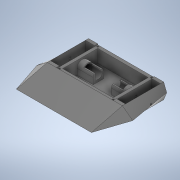
# Autodesk Inventor part: BodyWedgeV4
Saved by Autodesk Inventor 2020 (Build 240168000, 168)
## iProperties
Created: 2023-12-03
Part Number: BodyWedgeV4
Material: Thermoplastic Resin
Document SubType Name: Modeling
Designer: smz3rm
Density: 1.28 g/cm^3
Appearance: Smooth - Black
Mass: 334.957 g
Surface Area: 717.072 cm^2
Volume: 261.685 cm^3
Author: smz3rm
Autodesk Inventor part; units mm, degrees
ref_plane "YZ Plane" through (0, 0, 0) normal (1, 0, 0) x (0, 1, 0)
sketch "Sketch1" plane through (0, 0, 0) normal (0, 1, 0) x (-1, 0, 0)
  line L0 (55, 30) -> (-55, 30)
  line L1 (-55, 30) -> (-55, -30)
  line L2 (-55, -30) -> (55, -30)
  line L3 (55, -30) -> (55, 30)
  line L4 (55, 30) -> (-55, -30) construction
  line L5 (-55, 30) -> (55, -30) construction
  point P0 (0, 0)
  dimension "d0" = 110
  dimension "d1" = 60
  constraints: 12 end point, 2 midpoint, 2 parallel, 1 horizontal, 1 perpendicular
  measures "d0" distance of L2.end L1.end
  measures "d1" distance of L0.end L1.end
extrude "Extrusion1" add sketch "Sketch1" along normal blind 3
sketch "Sketch2" plane through (0, 3, 0) normal (0, 1, 0) x (1, 0, 0)
  line L0 (-55, 30) -> (-55, -30) projected
  line L1 (-55, -30) -> (55, -30) projected
  line L2 (55, -30) -> (55, 30) projected
  line L3 (55, 30) -> (-55, 30) projected
  line L4 (-49, 24) -> (-49, -24)
  line L5 (-49, -24) -> (49, -24)
  line L6 (49, -24) -> (49, 24)
  line L7 (49, 24) -> (-49, 24)
  point P0 (0, 0)
  dimension "d4" = 6
  constraints: 8 end point, 3 other
  measures "d4" distance between parallel lines of L3 L7
extrude "Extrusion2" add sketch "Sketch2" along normal blind 25.4125
sketch "Sketch3" plane through (-49, 3, 24) normal (1, 0, 0) x (0, 0, -1)
  line L0 (48, 0) -> (0, 0) projected
  line L1 (48, 0) -> (48, 25.4125) projected
  line L2 (0, 25.4125) -> (48, 25.4125) projected
  line L3 (0, 0) -> (0, 25.4125) projected
  circle A0 centre (38, 12) radius 8
  line L4 (54, -3) -> (-6, -3) projected
  circle A1 centre (38, 12) radius 10
  line L5 (48, 0) -> (48, 25.4125) projected
  line L6 (28, 12) -> (28, 0)
  point P0 (24, -3)
  point P1 (38, 22)
  point P2 (48, 12)
  dimension "d7" = 16
  dimension "d8" = 15
  dimension "d9" = 2
  constraints: 2 centre point, 2 end point, 2 point on circle, 2 tangent, 1 coincident, 1 point on line, 1 vertical
  measures "d7" diameter of A0
  measures "d8" distance from line of L4 A0.centre
  measures "d9" radial gap between concentric circles of A0 A1
extrude "Extrusion3" add sketch "Sketch3" along normal blind 11.25 contours L0 L6 A1 L1 | A1
sketch "Sketch4" plane through (-37.75, 3, 24) normal (1, 0, 0) x (0, 0, -1)
  line L0 (48, 12) -> (48, 0) projected
  arc A0 (48, 12) -> (28, 12) centre (38, 12) ccw projected
  line L1 (28, 12) -> (28, 0) projected
  line L2 (48, 0) -> (28, 0) projected
  circle A1 centre (38, 12) radius 8 projected
  circle A2 centre (38, 12) radius 7.75
  circle A3 centre (38, 12) radius 8 projected
  line L3 (48, 0) -> (28, 0) projected
  line L4 (32, 0) -> (32, 17.2915)
  line L5 (38, 19.75) -> (38, 4.25)
  line L6 (44, 0) -> (44, 17.2915)
  line L7 (32, 17.2915) -> (29.5147, 17.2915)
  arc A4 (48, 12) -> (28, 12) centre (38, 12) ccw projected
  line L8 (48, 12) -> (48, 0) projected
  line L9 (44, 17.2915) -> (46.4853, 17.2915)
  point P0 (24, -3)
  point P1 (48, 21)
  point P2 (39, 21)
  point P3 (44, 7.0946)
  point P4 (32, 7.0946)
  point P5 (44, 16.9054)
  point P6 (44, 0)
  point P7 (32, 16.9054)
  dimension "d13" = 15.5
  dimension "d14" = 15.5
  dimension "d15" = 12
  constraints: 10 end point, 4 point on circle, 2 horizontal, 2 symmetric about line, 1 centre point, 1 coincident, 1 perpendicular, 1 point on line, 1 vertical, 2 other
  measures "d13" diameter of A2
  measures "d14" distance of L5.start L5.end
  measures "d15" distance between parallel lines of L6 L4
extrude "Extrusion4" add sketch "Sketch4" along normal blind 20 contours L0 L2 L6 A1 L9 A0 | L2 L4 A1 L6 | L7 A1 L4 L2 L1 A0 | A1 L6 A2 | A1 L4 A2 L6 | L4 A2 A1 | L4 A2 picked at (37.1105, 4.2492)
sketch "Sketch13" plane through (-49, 15, -14) normal (1, 0, 0) x (0, 0, -1)
  circle A0 centre (0, 0) radius 2
  point P0 (-14, -15)
  dimension "d38" = 4
  constraints: 1 centre point
  measures "d38" diameter of A0
extrude "Extrusion13" cut sketch "Sketch13" against normal up to surface (6 mm away)
mirror "Mirror7" about plane through (0, 0, 0) normal (1, 0, 0) of "Extrusion3", "Extrusion4", "Extrusion13"
sketch "Sketch14" plane through (-55, 0, -30) normal (-1, 0, 0) x (0, 0, 1)
  circle A0 centre (16, 15) radius 2 projected
  line L0 (0, 0) -> (60, 0) projected
  line L1 (60, 0) -> (60, 28.4125) projected
  line L2 (0, 28.4125) -> (60, 28.4125) projected
  line L3 (0, 0) -> (0, 28.4125) projected
  line L4 (54, 28.4125) -> (54, 0)
  line L5 (0, 0) -> (60, 0) projected
  line L6 (54, 28.4125) -> (54, 30)
  line L7 (54, 30) -> (60, 30)
  line L8 (60, 30) -> (60, 28.4125)
  point P0 (30, 0)
  point P1 (54, 28.4125)
  point P2 (54, 28.4125)
  dimension "d74" = 1.5875
  constraints: 8 end point, 2 perpendicular, 2 vertical, 1 point on line
  measures "d74" distance of L4.start L6.end
extrude "Extrusion14" add sketch "Sketch14" along normal blind 17.78 contours L4 L2 L1 L0 | L6 L7 L8 L2
sketch "Sketch15" plane through (-55, 0, -30) normal (-1, 0, 0) x (0, 0, 1)
  line L0 (0, 28.4125) -> (54, 28.4125) projected
  line L1 (0, 0) -> (0, 28.4125) projected
  line L2 (0, 0) -> (54, 0) projected
  circle A0 centre (16, 15) radius 2 projected
  line L3 (0, 0) -> (0, 28.4125) projected
  line L4 (0, 28.4125) -> (-14, 28.4125)
  line L5 (-14, 28.4125) -> (-14, 0)
  line L6 (-14, 0) -> (0, 0)
  line L7 (54, 0) -> (54, 28.4125) projected
  point P0 (30, 0)
  dimension "d43" = 30
  constraints: 6 end point, 2 perpendicular, 1 horizontal
  measures "d43" distance from line of L5 A0.centre
extrude "Extrusion15" add sketch "Sketch15" against normal blind 6 contours L1 L6 L5 L4
sketch "Sketch16" plane through (0, 28.4125, 0) normal (0, 1, 0) x (1, 0, 0)
  line L0 (55, 30) -> (-49, 30) projected
  line L1 (-49, 44) -> (-49, 30) projected
  line L2 (-55, 44) -> (-49, 44) projected
  line L3 (-55, -24) -> (-55, 44) projected
  line L4 (-55, -30) -> (55, -30) projected
  line L5 (55, -30) -> (55, 30) projected
  line L6 (49, -24) -> (-49, -24) projected
  line L7 (-49, -24) -> (-49, 24) projected
  line L8 (-49, 24) -> (49, 24) projected
  line L9 (49, 24) -> (49, -24) projected
  line L10 (49, 24) -> (49, -24) projected
  line L11 (49, 24) -> (49, 30)
  line L12 (-49, 24) -> (49, 24) projected
  line L13 (55, 30) -> (-49, 30) projected
  line L14 (-49, 24) -> (-49, 30)
  line L15 (-55, -24) -> (-55, -30) projected
  point P0 (0, 0)
  constraints: 4 end point, 1 collinear, 1 point on line, 1 vertical
extrude "Extrusion16" cut sketch "Sketch16" against normal up to surface (25.4125 mm away) contours L11 L8 L14 L0
mirror "Mirror8" about plane through (0, 0, 0) normal (1, 0, 0) of "Extrusion15", "Extrusion14"
sketch "Sketch17" plane through (49, 0, -30) normal (0, 0, -1) x (-1, 0, 0)
  line L0 (0, 3) -> (0, 0) projected
  line L1 (0, 0) -> (98, 0) projected
  line L2 (98, 0) -> (98, 3) projected
  line L3 (98, 3) -> (0, 3) projected
  point P0 (49, 0)
extrude "Extrusion17" add sketch "Sketch17" along normal up to surface (14 mm away)
sketch "Sketch19" plane through (0, 0, 0) normal (0, -1, 0) x (1, 0, 0)
  line L0 (-55, -44) -> (-55, 24) projected
  line L1 (-55, -44) -> (55, -44) projected
  line L2 (55, 24) -> (55, -44) projected
  line L3 (72.78, 24) -> (72.78, 30) projected
  line L4 (72.78, 30) -> (-72.78, 30) projected
  line L5 (-72.78, 24) -> (-72.78, 30) projected
  line L6 (55, -44) -> (-55, -44)
  line L7 (-55, -44) -> (-55, -50)
  line L8 (-55, -50) -> (55, -50)
  line L9 (55, -50) -> (55, -44)
  line L10 (-55, -44) -> (-55, 24) projected
  line L11 (55, 24) -> (72.78, 24) projected
  line L12 (-55, 24) -> (-72.78, 24) projected
  point P0 (0, 0)
  dimension "d50" = 6
  constraints: 8 end point, 2 parallel, 1 collinear, 1 horizontal, 1 perpendicular
  measures "d50" distance of L7.end L6.end
extrude "Extrusion18" add sketch "Sketch19" against normal up to surface (28.4125 mm away) contours L1 L9 L8 L7
sketch "Sketch29" plane through (-55, 0, 24) normal (-1, 0, 0) x (0, 0, 1)
  line L0 (0, 0) -> (0, 28.4125) projected
  line L1 (0, 28.4125) -> (-74, 28.4125) projected
  line L2 (-74, 0) -> (-74, 28.4125) projected
  line L3 (-74, 0) -> (0, 0) projected
  circle A0 centre (-38, 15) radius 2 projected
  line L4 (-74, 0) -> (0, 0) projected
  line L5 (-68, 0) -> (-68, 30)
  line L6 (-68, 30) -> (-74, 30)
  line L7 (-74, 30) -> (-74, 28.4125)
  point P0 (-24, 0)
  point P1 (-68, 28.4125)
  dimension "d75" = 1.5875
  constraints: 6 end point, 2 perpendicular, 2 point on line, 1 horizontal
  measures "d75" distance from line of L1 L5.end
extrude "Extrusion25" add sketch "Sketch29" along normal up to surface (17.78 mm away) contours L3 L2 L1 L5 | L1 L7 L6 L5
sketch "Sketch31" plane through (-72.78, 0, -30) normal (-1, 0, 0) x (0, 0, 1)
  line L0 (54, 30) -> (54, 0) projected
  line L1 (54, 0) -> (60, 0) projected
  line L2 (60, 0) -> (60, 30) projected
  line L3 (60, 30) -> (54, 30) projected
  line L4 (60, 30) -> (120, 15)
  line L5 (60, 0) -> (60, 30) projected
  line L6 (120, 15) -> (60, 0)
  point P0 (30, 0)
  dimension "d78" = 60
  constraints: 4 end point, 1 equal length
  measures "d78" distance from line of L2 L4.end
sketch "Sketch32" plane through (-72.78, 30, 30) normal (0, 0, 1) x (1, 0, 0)
  line L0 (145.56, -30) -> (0, -30) projected
  line L1 (145.56, -30) -> (145.56, 0) projected
  line L2 (127.78, 0) -> (145.56, 0) projected
  line L3 (127.78, -1.5875) -> (127.78, 0) projected
  line L4 (17.78, -1.5875) -> (127.78, -1.5875) projected
  line L5 (17.78, -1.5875) -> (17.78, 0) projected
  line L6 (17.78, 0) -> (0, 0) projected
  line L7 (0, -30) -> (0, 0) projected
  line L8 (0, 0) -> (-20, -15)
  line L9 (17.78, -30) -> (0, -30) projected
  line L10 (-20, -15) -> (0, -30)
  point P0 (72.78, -30)
  dimension "d79" = 20
  constraints: 4 end point, 1 equal length
  measures "d79" distance from line of L7 L8.end
extrude "Extrusion26" add sketch "Sketch31" against normal up to surface (145.56 mm away) contours L4 L6 L2
extrude "Extrusion27" add sketch "Sketch32" along normal up to surface (60 mm away) contours L10 L8 L7
ref_plane "Work Plane9" through (-72.78, 30, 30) normal (0.5883484, -0.7844645, -0.1961161) x (0, -0.2425356, 0.9701425)
sketch "Sketch33" plane through (-72.78, 30, 30) normal (0.5883484, -0.7844645, -0.1961161) x (0, -0.2425356, 0.9701425)
  line L0 (-26.0298, -27.3622) -> (95.8172, -27.3622)
  line L1 (95.8172, -27.3622) -> (95.8172, 41.2642)
  line L2 (95.8172, 41.2642) -> (-26.0298, 41.2642)
  line L3 (-26.0298, 41.2642) -> (-26.0298, -27.3622)
  point P0 (-21.8282, -37.4461)
  constraints: 8 end point, 2 parallel, 1 horizontal, 1 perpendicular
ref_plane "Work Plane10" through (-72.78, 0, 30) normal (-0.5883484, -0.7844645, 0.1961161) x (0, 0.2425356, 0.9701425)
sketch "Sketch34" plane through (-72.78, 0, 30) normal (-0.5883484, -0.7844645, 0.1961161) x (0, 0.2425356, 0.9701425)
  line L0 (-38.3211, 46.7745) -> (150.818, 46.7745)
  line L1 (150.818, 46.7745) -> (150.818, -38.4713)
  line L2 (150.818, -38.4713) -> (-38.3211, -38.4713)
  line L3 (-38.3211, -38.4713) -> (-38.3211, 46.7745)
  point P0 (-29.1043, -54.5696)
  constraints: 8 end point, 2 parallel, 1 horizontal, 1 perpendicular
extrude "Extrusion28" cut sketch "Sketch33" against normal through all
extrude "Extrusion29" cut sketch "Sketch34" along normal through all
sketch "Sketch35" plane through (-72.78, 30, 30) normal (0, 0, -1) x (-1, 0, 0)
  line L0 (0, -30) -> (0, 0) projected
  line L1 (20, -15) -> (0, -30) projected
  line L2 (0, 0) -> (20, -15) projected
  point P0 (-72.78, -30)
sketch "Sketch36" plane through (55, 0, -50) normal (0, 0, -1) x (-1, 0, 0)
  line L0 (110, 30) -> (127.78, 30) projected
  line L1 (127.78, 30) -> (133.78, 15)
  line L2 (133.78, 15) -> (127.78, 0)
  line L3 (127.78, 0) -> (127.78, 30) projected
  point P0 (55, 0)
  dimension "d88" = 6
  constraints: 4 end point, 1 equal length
  measures "d88" distance from line of L3 L1.end
loft "Loft2" add profiles "Sketch35", "Sketch36"
sketch "Sketch37" plane through (-55, 0, 24) normal (-1, 0, 0) x (0, 0, 1)
  circle A0 centre (-38, 15) radius 2 projected
  line L0 (-68, 28.4125) -> (-68, 0) projected
  line L1 (-68, 0) -> (0, 0) projected
  line L2 (0, 0) -> (0, 28.4125) projected
  line L3 (0, 28.4125) -> (-68, 28.4125) projected
  point P0 (-24, 0)
extrude "Extrusion30" cut sketch "Sketch37" along normal through all contours A0
mirror "Mirror11" about plane through (0, 0, 0) normal (1, 0, 0) of "Extrusion30", "Loft2", "Extrusion29", "Extrusion28", "Extrusion27", "Extrusion25"
sketch "Sketch38" plane through (0, 28.4125, 0) normal (0, 1, 0) x (1, 0, 0)
  line L0 (49, 44) -> (49, -24) projected
  line L1 (49, -24) -> (-49, -24) projected
  line L2 (-49, -24) -> (-49, 44) projected
  line L3 (49, 44) -> (-49, 44) projected
  line L4 (55, -24) -> (55, 44) projected
  line L5 (55, 44) -> (55, 50) projected
  line L6 (-55, 50) -> (55, 50) projected
  line L7 (-55, 44) -> (-55, 50) projected
  line L8 (-55, -24) -> (-55, 44) projected
  line L9 (-55, -24) -> (-55, -30) projected
  line L10 (-55, -30) -> (55, -30) projected
  line L11 (55, -30) -> (55, -24) projected
  line L12 (55, -30) -> (55, -24) projected
  line L13 (55, -27) -> (-55, -27)
  line L14 (-55, -30) -> (55, -30) projected
  line L15 (-52, -30) -> (-52, 50)
  line L16 (-55, 50) -> (55, 50) projected
  line L17 (55, 44) -> (55, 50) projected
  line L18 (55, 47) -> (-55, 47)
  circle A0 centre (-52, -27) radius 1.4
  circle A1 centre (-52, 47) radius 1.4
  point P0 (0, 0)
  dimension "d95" = 3
  dimension "d96" = 2.8
  dimension "d97" = 2.8
  constraints: 6 end point, 6 point on line, 4 midpoint, 2 centre point, 1 perpendicular
  measures "d95" distance of L6.start L15.end
  measures "d96" diameter of A0
  measures "d97" diameter of A1
extrude "Extrusion31" cut sketch "Sketch38" against normal blind 6 contours A0 L15 L13 | L13 L15 A0 | A1 L15 L18 | L18 L15 A1 | L15 A0 L13 | L13 A0 L15 | L18 A1 L15 | L15 A1 L18
mirror "Mirror12" about plane through (0, 0, 0) normal (1, 0, 0) of "Extrusion31"
equation "\"d0\" = BoxWidth"
equation "\"d1\" = BoxLength"
equation "\"d2\" = BaseThickness"
equation "\"d4\" = SideThickness"
equation "\"d5\" = -BaseThickness + Height - TopThickness"
equation "\"d8\" = MotorHeight"
equation "\"d9\" = MotorMountThickness"
equation "\"d39\" = ForkLength"
equation "\"d74\" = TopThickness"
equation "\"d41\" = WheelWidth"
equation "\"d44\" = SideThickness"
equation "\"d50\" = SideThickness"
equation "\"d75\" = TopThickness"
equation "\"d76\" = WheelWidth"
equation "\"d78\" = ForkLength"
equation "\"d79\" = WedgeWidth"
equation "\"d80\" = WheelWidth"
equation "\"d82\" = WheelWidth"
equation "\"d88\" = SideThickness"
equation "\"d95\" = 0.5 * SideThickness"
equation "\"d96\" = ScrewDia"
equation "\"d97\" = ScrewDia"
equation "\"d98\" = ScrewDepth"
equation "\"WedgeWidth\" = 20"
equation "\"Height\" = 30"
equation "\"BoxLength\" = 60"
equation "\"SideThickness\" = 6"
equation "\"BaseThickness\" = 3"
equation "\"BoxWidth\" = 110"
equation "\"WheelWidth\" = 17.78"
equation "\"ForkLength\" = 60"
equation "\"TopThickness\" = 1.5875"
equation "\"SideTriangleWidth\" = 15"
equation "\"MotorHeight\" = 0.5 * Height"
equation "\"MotorMountThickness\" = 2"
equation "\"WheelDia\" = 57.15"
equation "\"ScrewDia\" = 2.8"
equation "\"ScrewDepth\" = 6"
body "Solid1"
